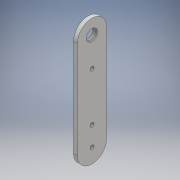
# Autodesk Inventor part: BaseJoint
Saved by Autodesk Inventor 2018 (Build 220112000, 112)
## iProperties
Created: 2017-05-30
Part Number: BaseJoint
Material: Generic
Document SubType Name: Modeling
Designer: Damian
Density: 1 g/cm^3
Appearance: Default
Author: Damian
Autodesk Inventor part; units mm, degrees
ref_plane "YZ Plane" through (0, 0, 0) normal (1, 0, 0) x (0, 1, 0)
ref_plane "XZ Plane" through (0, 0, 0) normal (0, 1, 0) x (-1, 0, 0)
ref_plane "XY Plane" through (0, 0, 0) normal (0, 0, 1) x (1, 0, 0)
sketch "Sketch1" plane through (0, 0, 0) normal (1, 0, 0) x (0, 1, 0)
  arc A0 (43.0231, 66.0406) -> (13.0231, 66.0406) centre (28.0231, 66.0406) ccw
  arc A1 (13.0231, -33.9594) -> (43.0231, -33.9594) centre (28.0231, -33.9594) ccw
  line L0 (13.0231, 66.0406) -> (13.0231, -33.9594)
  line L1 (43.0231, 66.0406) -> (43.0231, -33.9594)
  circle A2 centre (28.0231, 66.0406) radius 5
  circle A3 centre (28.0231, -33.9594) radius 2
  circle A4 centre (28.0231, 36.0406) radius 2
  circle A5 centre (28.0231, -13.9594) radius 2
  point P0 (0, 0)
  dimension "d6" = 15
  dimension "d18" = 100
  dimension "d40" = 10
  dimension "d50" = 0
  dimension "d51" = 0
  dimension "d52" = 20
  dimension "d53" = 30
  dimension "d54" = 4
  constraints: 6 centre point, 4 end point, 4 point on circle, 4 tangent, 2 coincident, 2 vertical, 1 equal radius
  measures "d6" radius of A1
  measures "d18" distance of A1.centre A0.centre
  measures "d40" diameter of A2
  measures "d50" horizontal distance of A0.centre A4.centre
  measures "d51" horizontal distance of A4.centre A5.centre
  measures "d52" distance of A1.centre A5.centre
  measures "d53" distance of A0.centre A4.centre
  measures "d54" diameter of A5
extrude "Extrusion6" add sketch "Sketch1" along normal blind 4
hole "Hole4" at (4, 28.0231, 66.0406) direction (-1, 0, 0) diameter 11.6 depth 0.8 tip angle 118
body "Solid2"
